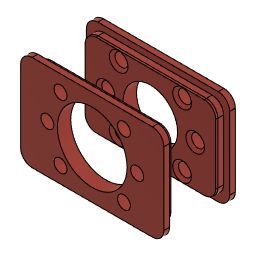
2010 Ballscrew Plates (Autodesk Fusion 360 design; units mm, degrees)
Autodesk Fusion 360 part; units mm, degrees
sketch "Sketch1" plane through (0, 0, 0) normal (0, 1, 0) x (1, 0, 0) in component "2010 Ballscrew Plate"
  line L0 (0, 0) -> (75, 0)
  line L1 (75, 0) -> (75, -50)
  line L2 (75, -50) -> (0, -50)
  line L3 (0, -50) -> (0, 0)
  dimension "d5" = 75
  dimension "d6" = 50
  constraint horizontal L0
  constraint vertical L1
  constraint horizontal L2
  constraint vertical L3
  constraint coincident L0.start L3.end
  measures "d5" distance of L0.start L0.end
  measures "d6" distance of L0.start L2.end
extrude "Extrude1" add sketch "Sketch1" along normal blind 3 makes body 1 in component "2010 Ballscrew Plate"
sketch "Sketch2" plane through (0, 3, 0) normal (0, 1, 0) x (-1, 0, 0) in component "2010 Ballscrew Plate"
  line L0 (0, 50) -> (-75, 50)
  line L1 (-75, 50) -> (-75, 0)
  line L2 (-75, 0) -> (0, 0)
  line L3 (0, 0) -> (0, 50)
  line L4 (-75, 50) -> (0, 0) construction
  line L5 (-3.15, 46.85) -> (-71.85, 46.85)
  line L6 (-71.85, 46.85) -> (-71.85, 3.15)
  line L7 (-71.85, 3.15) -> (-3.15, 3.15)
  line L8 (-3.15, 3.15) -> (-3.15, 46.85)
  line L9 (-3.15, 46.85) -> (-71.85, 3.15) construction
  line L10 (-71.85, 46.85) -> (-3.15, 3.15) construction
  point P0 (-37.5, 25)
  dimension "d9" = 68.7
  dimension "d10" = 43.7
  constraint coincident L0.end L1.start
  constraint coincident L2.end L3.start
  constraint horizontal L5
  constraint perpendicular L5 L6
  constraint parallel L5 L7
  constraint parallel L6 L8
  constraint coincident L9 P0
  constraint coincident L10 P0
  constraint midpoint L4 P0
  measures "d9" distance of L6.end L7.end
  measures "d10" distance of L5.end L6.end
extrude "Extrude2" add sketch "Sketch2" along normal blind 4 contours L5 L6 L7 L8 bodies 1 in component "2010 Ballscrew Plate"
sketch "Sketch3" plane through (0, 7, 0) normal (0, 1, 0) x (-1, 0, 0) in component "2010 Ballscrew Plate"
  line L0 (-3.15, 3.15) -> (-3.15, 46.85)
  line L1 (-3.15, 46.85) -> (-71.85, 46.85)
  line L2 (-71.85, 46.85) -> (-71.85, 3.15)
  line L3 (-71.85, 3.15) -> (-3.15, 3.15)
  line L4 (-71.85, 46.85) -> (-3.15, 3.15) construction
  circle A0 centre (-37.5, 25) radius 18.25
  line L5 (-37.5, 25) -> (-14, 25) construction
  line L6 (-37.5, 25) -> (-61, 25) construction
  circle A1 centre (-61, 25) radius 3.4
  circle A2 centre (-14, 25) radius 3.4
  circle A3 centre (-20.883, 41.617) radius 3.4
  circle A4 centre (-54.117, 8.383) radius 3.4
  circle A5 centre (-54.117, 41.617) radius 3.4
  circle A6 centre (-20.883, 8.383) radius 3.4
  circle A7 centre (-61, 25) radius 3.4
  circle A8 centre (-14, 25) radius 3.4
  dimension "d13" = 36.5
  dimension "d14" = 23.5
  dimension "d15" = 23.5
  dimension "d16" = 6.8
  dimension "d17" = 6.8
  dimension "d19" = 180
  constraint coincident L1.end L2.start
  constraint coincident L0.start L3.end
  constraint midpoint L4 A0.centre
  constraint coincident A0.centre L5.start
  constraint horizontal L5
  constraint parallel L5 L6
  constraint coincident L6.end A1.centre
  constraint coincident L5.end A2.centre
  measures "d13" diameter of A0
  measures "d14" distance of A0.centre L5.end
  measures "d15" distance of A0.centre L6.end
  measures "d16" diameter of A1
  measures "d17" diameter of A2
extrude "Extrude3" cut sketch "Sketch3" against normal through all contours A0 | A1 A7 | A2 A8 | A3 | A4 | A5 | A6 bodies 1 in component "2010 Ballscrew Plate"
fillet "Fillet1" radius 6 8 edges at (71.85, 5, 46.85) (75, 1.5, 50) (0, 1.5, 50) (3.15, 5, 46.85) (3.15, 5, 3.15) (0, 1.5, 0) (75, 1.5, 0) (71.85, 5, 3.15) on bodies 1 in component "2010 Ballscrew Plate"
sketch "Sketch1 (2)" plane through (0, 0, 0) normal (0, 1, 0) x (1, 0, 0) in component "2010 Ballscrew Plate (Chamfered)"
  line L0 (0, 0) -> (75, 0)
  line L1 (75, 0) -> (75, -50)
  line L2 (75, -50) -> (0, -50)
  line L3 (0, -50) -> (0, 0)
  dimension "d5_1" = 75
  dimension "d6_1" = 50
  constraint horizontal L0
  constraint vertical L1
  constraint horizontal L2
  constraint vertical L3
  constraint coincident L0.start L3.end
  measures "d5_1" distance of L0.start L0.end
  measures "d6_1" distance of L0.start L2.end
extrude "Extrude1'" add sketch "Sketch1 (2)" along normal blind 3 separate body makes body 2 in component "2010 Ballscrew Plate (Chamfered)"
sketch "Sketch2 (2)" plane through (0, 3, 0) normal (0, 1, 0) x (-1, 0, 0) in component "2010 Ballscrew Plate (Chamfered)"
  line L0 (0, 50) -> (-75, 50)
  line L1 (-75, 50) -> (-75, 0)
  line L2 (-75, 0) -> (0, 0)
  line L3 (0, 0) -> (0, 50)
  line L4 (-75, 50) -> (0, 0) construction
  line L5 (-3.15, 46.85) -> (-71.85, 46.85)
  line L6 (-71.85, 46.85) -> (-71.85, 3.15)
  line L7 (-71.85, 3.15) -> (-3.15, 3.15)
  line L8 (-3.15, 3.15) -> (-3.15, 46.85)
  line L9 (-3.15, 46.85) -> (-71.85, 3.15) construction
  line L10 (-71.85, 46.85) -> (-3.15, 3.15) construction
  point P0 (-37.5, 25)
  dimension "d9_1" = 68.7
  dimension "d10_1" = 43.7
  constraint coincident L0.end L1.start
  constraint coincident L2.end L3.start
  constraint horizontal L5
  constraint perpendicular L5 L6
  constraint parallel L5 L7
  constraint parallel L6 L8
  constraint coincident L9 P0
  constraint coincident L10 P0
  constraint midpoint L4 P0
  measures "d9_1" distance of L6.end L7.end
  measures "d10_1" distance of L5.end L6.end
extrude "Extrude2'" add sketch "Sketch2 (2)" along normal blind 4 contours L5 L6 L7 L8 bodies 2 in component "2010 Ballscrew Plate (Chamfered)"
sketch "Sketch3 (2)" plane through (0, 7, 0) normal (0, 1, 0) x (-1, 0, 0) in component "2010 Ballscrew Plate (Chamfered)"
  line L0 (-3.15, 3.15) -> (-3.15, 46.85)
  line L1 (-3.15, 46.85) -> (-71.85, 46.85)
  line L2 (-71.85, 46.85) -> (-71.85, 3.15)
  line L3 (-71.85, 3.15) -> (-3.15, 3.15)
  line L4 (-71.85, 46.85) -> (-3.15, 3.15) construction
  circle A0 centre (-37.5, 25) radius 14.25
  line L5 (-37.5, 25) -> (-14, 25) construction
  line L6 (-37.5, 25) -> (-61, 25) construction
  circle A1 centre (-61, 25) radius 3.4
  circle A2 centre (-14, 25) radius 3.4
  circle A3 centre (-20.883, 41.617) radius 3.4
  circle A4 centre (-54.117, 8.383) radius 3.4
  circle A5 centre (-54.117, 41.617) radius 3.4
  circle A6 centre (-20.883, 8.383) radius 3.4
  circle A7 centre (-61, 25) radius 3.4
  circle A8 centre (-14, 25) radius 3.4
  dimension "d13_1" = 28.5
  dimension "d14_1" = 23.5
  dimension "d15_1" = 23.5
  dimension "d16_1" = 6.8
  dimension "d17_1" = 6.8
  dimension "d19_1" = 180
  constraint coincident L1.end L2.start
  constraint coincident L0.start L3.end
  constraint midpoint L4 A0.centre
  constraint coincident A0.centre L5.start
  constraint horizontal L5
  constraint parallel L5 L6
  constraint coincident L6.end A1.centre
  constraint coincident L5.end A2.centre
  measures "d13_1" diameter of A0
  measures "d14_1" distance of A0.centre L5.end
  measures "d15_1" distance of A0.centre L6.end
  measures "d16_1" diameter of A1
  measures "d17_1" diameter of A2
extrude "Extrude3'" cut sketch "Sketch3 (2)" against normal through all contours A0 | A1 A7 | A2 A8 | A3 | A4 | A5 | A6 bodies 2 in component "2010 Ballscrew Plate (Chamfered)"
fillet "Fillet1'" radius 6 8 edges at (71.85, 5, 46.85) (75, 1.5, 50) (0, 1.5, 50) (3.15, 5, 46.85) (3.15, 5, 3.15) (0, 1.5, 0) (75, 1.5, 0) (71.85, 5, 3.15) on bodies 2 in component "2010 Ballscrew Plate (Chamfered)"
chamfer "Chamfer1" distance 1.5 angle 45 6 edges at (57.2869, 7, 42.8465) (64.1699, 7, 26.2295) (57.2869, 7, 9.6125) (24.0529, 7, 9.6125) (17.1699, 7, 26.2295) (24.0529, 7, 42.8465) on bodies 2 in component "2010 Ballscrew Plate (Chamfered)"
chamfer "Chamfer2" distance 1 angle 10 8 edges at (70.0926, 7, 45.0926) (71.85, 7, 25) (70.0926, 7, 4.9074) (37.5, 7, 3.15) (4.9074, 7, 4.9074) (3.15, 7, 25) (4.9074, 7, 45.0926) (37.5, 7, 46.85) measured on face at (68.85, 4.3333, 46.0462) measured on face at (64.3906, 7, 36.6341) measured on face at (68.85, 5.6667, 3.9538) measured on face at (64.3906, 7, 36.6341) measured on face at (8.8645, 4.3333, 3.1568) measured on face at (64.3906, 7, 36.6341) measured on face at (8.8645, 4.3333, 46.8432) measured on face at (64.3906, 7, 36.6341) on bodies 2 in component "2010 Ballscrew Plate (Chamfered)"
chamfer "Chamfer1'" distance 1 angle 10 8 edges at (70.0926, 7, 45.0926) (71.85, 7, 25) (70.0926, 7, 4.9074) (37.5, 7, 3.15) (4.9074, 7, 4.9074) (3.15, 7, 25) (4.9074, 7, 45.0926) (37.5, 7, 46.85) measured on face at (68.85, 4.3333, 46.0462) measured on face at (63.7575, 7, 36.3856) measured on face at (68.85, 5.6667, 3.9538) measured on face at (63.7575, 7, 36.3856) measured on face at (8.8645, 4.3333, 3.1568) measured on face at (63.7575, 7, 36.3856) measured on face at (8.8645, 4.3333, 46.8432) measured on face at (63.7575, 7, 36.3856) on bodies 1 in component "2010 Ballscrew Plate"
component "2010 Ballscrew Plate" placed x (1, 0, 0) y (0, 1, 0) z (0, 0, 1) at (0, 0, 0)
component "2010 Ballscrew Plate (Chamfered)" placed x (1, 0, 0) y (0, 1, 0) z (0, 0, 1) at (0, 0, 0)
equation "extrusionTall = 75 mm"
equation "extrusionNarrow = 50 mm"
equation "extrusionRadius = 6 mm"
equation "extrusionThickness = 3 mm"
equation "d5 = extrusionTall"
equation "d6 = extrusionNarrow"
equation "d9 = extrusionTall - ( 2 * extrusionThickness ) - 0.3 mm"
equation "d10 = extrusionNarrow - ( 2 * extrusionThickness ) - 0.3 mm"
equation "d14 = ( 47 / 2 ) * 1 mm"
equation "d15 = ( 47 / 2 ) * 1 mm"
equation "d22 = extrusionRadius"
equation "d5_1 = extrusionTall"
equation "d6_1 = extrusionNarrow"
equation "d9_1 = extrusionTall - ( 2 * extrusionThickness ) - 0.3 mm"
equation "d10_1 = extrusionNarrow - ( 2 * extrusionThickness ) - 0.3 mm"
equation "d14_1 = ( 47 / 2 ) * 1 mm"
equation "d15_1 = ( 47 / 2 ) * 1 mm"
equation "d22_1 = extrusionRadius"
